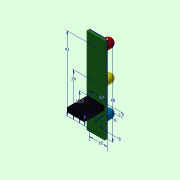
# Autodesk Inventor part: Led_Board_V1
Saved by Autodesk Inventor 2016 (Build 200138000, 138)
## iProperties
Created: 2014-12-24
Part Number: Led_Board_V1
Material: Generic
Document SubType Name: Modeling
Designer: Openlab
Density: 1 g/cm^3
Appearance: Smooth - Dark Forest Green
Mass: 2.60407 g
Surface Area: 31.9711 cm^2
Volume: 2.60407 cm^3
Author: Openlab
Autodesk Inventor part; units mm, degrees
ref_plane "YZ Plane" through (0, 0, 0) normal (1, 0, 0) x (0, 1, 0)
ref_plane "XZ Plane" through (0, 0, 0) normal (0, 1, 0) x (-1, 0, 0)
ref_plane "XY Plane" through (0, 0, 0) normal (0, 0, 1) x (1, 0, 0)
sketch "Sketch1" plane through (0, 0, 0) normal (0, 1, 0) x (-1, 0, 0)
  line L0 (10, 0) -> (0, 0)
  line L1 (0, 0) -> (0, -48)
  line L2 (0, -48) -> (10, -48)
  line L3 (10, -48) -> (10, 0)
  circle A0 centre (5, -7) radius 2.5
  circle A1 centre (5, -24) radius 2.5
  circle A2 centre (5, -41) radius 2.5
  circle A3 centre (5, -7) radius 3
  circle A4 centre (5, -24) radius 3
  circle A5 centre (5, -41) radius 3
  line L4 (5, -16) -> (5, -46.75) construction
  line L5 (9.75, -33.75) -> (0.25, -33.75)
  line L6 (0.25, -31.25) -> (9.75, -31.25)
  line L7 (6.1849, -32.5) -> (1.6849, -32.5) construction
  line L8 (9.75, -31.25) -> (9.75, -33.75)
  line L9 (0.25, -31.25) -> (0.25, -33.75)
  dimension "d0" = 48
  dimension "d1" = 10
  dimension "d4" = 5
  dimension "d24" = 6
  dimension "d48" = 7
  dimension "d49" = 24
  dimension "d50" = 41
  dimension "d51" = 2.5
  dimension "d52" = 15.5
  dimension "d53" = 9.5
  constraints: 20 end point, 6 centre point, 4 coincident, 4 equal radius, 4 perpendicular, 2 horizontal, 2 parallel, 2 vertical, 2 vertical alignment, 1 point on line, 3 other
  measures "d0" distance of L0.end L1.end
  measures "d1" distance of L1.end L2.end
  measures "d4" diameter of A2
  measures "d24" diameter of A5
  measures "d48" distance from line of L2 A2.centre
  measures "d49" distance from line of A1.centre L2
  measures "d50" distance from line of A0.centre L2
  measures "d51" distance between parallel lines of L5 L6
  measures "d52" distance between parallel lines of L2 L7
  measures "d53" distance between parallel lines of L9 L8
extrude "Extrusion1" add sketch "Sketch1" against normal blind 1.4 contours L3 L2 L1 L0 | A0 | A1 | A2 | A3 | A4 | A5 | L5 L9 L6 L8
extrude "Extrusion5" add sketch "Sketch1" along normal blind 8 contours A0
extrude "Extrusion6" add sketch "Sketch1" along normal blind 1 contours A3
fillet "Fillet4" radius 2.5 1 edges at (-2.5, 8, -7)
extrude "Extrusion7" add sketch "Sketch1" along normal blind 1 contours A4
extrude "Extrusion8" add sketch "Sketch1" along normal blind 8 contours A1
fillet "Fillet5" radius 2.5 1 edges at (-2.5, 8, -24)
extrude "Extrusion9" add sketch "Sketch1" along normal blind 8 contours A2
extrude "Extrusion10" add sketch "Sketch1" along normal blind 1 contours A5
fillet "Fillet6" radius 2.5 1 edges at (-2.5, 8, -41)
sketch "Sketch2" plane through (-5, 8, -24) normal (0, 1, 0) x (1, 0, 0)
  point P0 (0, 0)
extrude "Extrusion11" add sketch "Sketch1" against normal blind 12.5 contours L5 L9 L6 L8
body "Solid1"
